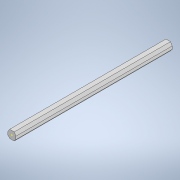
# Autodesk Inventor part: pillar
Saved by Autodesk Inventor 2022 (Build 260153000, 153)
## iProperties
Created: 2021-07-26
Part Number: pillar
Material: Generic
Document SubType Name: Modeling
Designer: DELL
Density: 1 g/cm^3
Appearance: Default
Author: DELL
Autodesk Inventor part; units mm, degrees
ref_plane "YZ Plane" through (0, 0, 0) normal (1, 0, 0) x (0, 1, 0)
ref_plane "XZ Plane" through (0, 0, 0) normal (0, 1, 0) x (-1, 0, 0)
ref_plane "XY Plane" through (0, 0, 0) normal (0, 0, 1) x (1, 0, 0)
sketch "Sketch1" plane through (0, 0, 0) normal (0, 0, 1) x (1, 0, 0)
  line L0 (3.7307, 6.0592) -> (-3.572, 6.0592)
  line L1 (-3.572, 6.0592) -> (-6.5354, 1.4553)
  line L2 (-6.5354, 1.4553) -> (-6.5354, -3.2545)
  line L3 (-6.5354, -3.2545) -> (-3.572, -6.6413)
  line L4 (-3.572, -6.6413) -> (3.7307, -6.6413)
  line L5 (3.7307, 6.0592) -> (6.4435, 1.4553)
  line L6 (6.4435, 1.4553) -> (6.4435, -3.2545)
  line L7 (6.4435, -3.2545) -> (3.7307, -6.6413)
  point P0 (0, 0)
  constraints: 16 end point, 1 horizontal, 1 parallel, 1 perpendicular, 1 vertical
extrude "Extrusion1" add sketch "Sketch1" along normal blind 250
sketch "Sketch2" plane through (0, 0, 250) normal (0, 0, 1) x (1, 0, 0)
  point P0 (0, 0)
body "Solid1"
